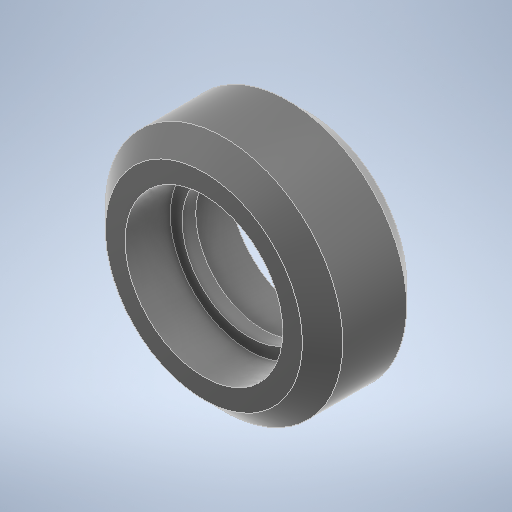
# Autodesk Inventor part: Rollers
Saved by Autodesk Inventor 2025 (Build 290162000, 162)
## iProperties
Manager: J. Wilburn
Created: 2025-03-12
Part Number: Rollers
Material: Acetal Resin, Black
Document SubType Name: Modeling
Designer: MAL16204
Density: 1.425 g/cm^3
Appearance: Smooth - Black
Description: Ball bearing rollers
Mass: 3.52812 g
Surface Area: 17.5146 cm^2
Volume: 2.47587 cm^3
Author: Richard Malstrom
Title: Rollers
Subject: Ender 3 Pro Assembly
Autodesk Inventor part; units mm, degrees
ref_plane "YZ Plane" through (0, 0, 0) normal (1, 0, 0) x (0, 1, 0)
ref_plane "XZ Plane" through (0, 0, 0) normal (0, 1, 0) x (-1, 0, 0)
ref_plane "XY Plane" through (0, 0, 0) normal (0, 0, 1) x (1, 0, 0)
sketch "Sketch1" plane through (0, 0, 0) normal (0, 0, 1) x (1, 0, 0)
  circle A0 centre (0, 0) radius 6.8
  circle A1 centre (0, 0) radius 12.05
  dimension "d10" = 13.6
  dimension "d11" = 24.1
  constraints: 2 centre point, 1 coincident
  measures "d10" diameter of A0
  measures "d11" diameter of A1
extrude "Extrusion3" add sketch "Sketch1" along normal mid plane 1.38
sketch "Sketch2" plane through (0, 0, 0) normal (0, 0, 1) x (1, 0, 0)
  circle A0 centre (0, 0) radius 12.05
  circle A1 centre (0, 0) radius 8
  dimension "d14" = 24.1
  dimension "d15" = 16
  constraints: 2 centre point, 2 coincident
  measures "d14" diameter of A0
  measures "d15" diameter of A1
extrude "Extrusion4" add sketch "Sketch2" along normal mid plane 10.58
chamfer "Chamfer2" distance 2.05 angle 45 2 edges at (-12.05, 0, 5.29) (-12.05, 0, -5.29)
body "Solid2"
